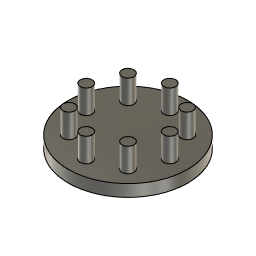
Intro to 2D Sketching and Constraints (Autodesk Fusion 360 design; units mm, degrees)
Autodesk Fusion 360 part; units mm, degrees
sketch "Sketch1" plane through (0, 0, 0) normal (0, 0, 1) x (1, 0, 0)
  line L0 (0, 0) -> (-175, 0) construction
  circle A0 centre (0, 0) radius 250
  circle A1 centre (-175, 0) radius 25
  circle A2 centre (-123.7437, -123.7437) radius 25
  circle A3 centre (0, -175) radius 25
  circle A4 centre (123.7437, -123.7437) radius 25
  circle A5 centre (175, 0) radius 25
  circle A6 centre (123.7437, 123.7437) radius 25
  circle A7 centre (0, 175) radius 25
  circle A8 centre (-123.7437, 123.7437) radius 25
  dimension "d32" = 175
  dimension "d33" = 500
  dimension "d34" = 50
  dimension "d36" = 360
  constraint coincident L0.start A0.centre
  constraint horizontal L0
  constraint coincident L0.end A1.centre
  measures "d32" distance of L0.start L0.end
  measures "d33" diameter of A0
  measures "d34" diameter of A1
extrude "Extrude1" add sketch "Sketch1" along normal blind 150 contours A1 | A2 | A3 | A4 | A5 | A6 | A7 | A8 makes body 1 at (24.9689, -176.2461, 100) makes body 2 at (24.9689, 173.7539, 100) makes body 3 at (148.7126, 122.4975, 100) makes body 4 at (-98.7748, -124.9898, 100) makes body 5 at (148.7126, -124.9898, 100) makes body 6 at (-98.7748, 122.4975, 100) makes body 7 at (199.9689, -1.2461, 100) makes body 8 at (-150.0311, -1.2461, 100)
extrude "Extrude2" add sketch "Sketch1" along normal blind 50 bodies 1 2 3 4 5 6 7 8
